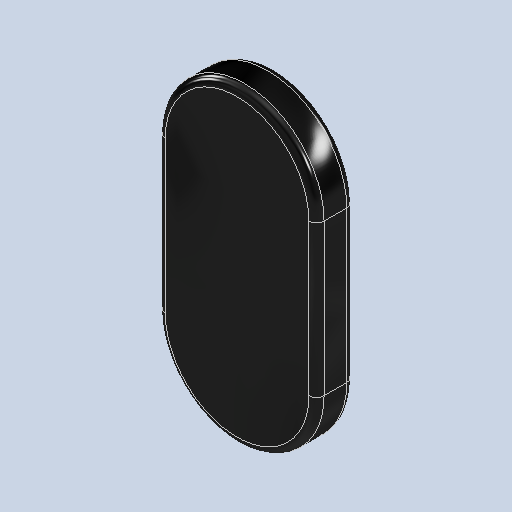
# Autodesk Inventor part: Feets
Saved by Autodesk Inventor 2023.1 (Build 271208000, 208)
## iProperties
Created: 2022-09-12
Part Number: Feets
Material: Generisch
Document SubType Name: Modeling
Designer: Rama
Density: 1 g/cm^3
Appearance: Schwarz
Author: Rama
Autodesk Inventor part; units mm, degrees
ref_plane "YZ Plane" through (0, 0, 0) normal (1, 0, 0) x (0, 1, 0)
ref_plane "XZ Plane" through (0, 0, 0) normal (0, 1, 0) x (-1, 0, 0)
ref_plane "XY Plane" through (0, 0, 0) normal (0, 0, 1) x (1, 0, 0)
sketch "Skizze1" plane through (0, 0, 0) normal (0, 0, 1) x (1, 0, 0)
  arc A0 (3.65, -3.2996) -> (8.25, -3.2996) centre (5.95, -3.2996) ccw projected
  line L0 (8.25, 0.7004) -> (8.25, -3.2996) projected
  arc A1 (8.25, 0.7004) -> (3.65, 0.7004) centre (5.95, 0.7004) ccw projected
  line L1 (3.65, -3.2996) -> (3.65, 0.7004) projected
  line L2 (5.95, -3.2996) -> (5.95, 0.7004) construction
  line L3 (8.05, -3.2996) -> (8.05, 0.7004)
  line L4 (3.85, 0.7004) -> (3.85, -3.2996)
  arc A2 (3.85, -3.2996) -> (8.05, -3.2996) centre (5.95, -3.2996) ccw
  arc A3 (8.05, 0.7004) -> (3.85, 0.7004) centre (5.95, 0.7004) ccw
  point P0 (0, 0)
  point P1 (5.95, -1.2996)
  dimension "d0" = 4.2
  constraints: 8 end point, 4 point on circle, 4 tangent, 2 centre point, 1 midpoint, 1 parallel, 1 vertical
  measures "d0" diameter of A3
extrude "Extrusion1" add sketch "Skizze1" along normal blind 1 contours A2 L4 A3 L3
fillet "Rundung1" radius 0.2 8 edges at (5.95, 2.8004, 1) (3.85, -1.2996, 1) (5.95, -5.3996, 1) (8.05, -1.2996, 1) (5.95, 2.8004, 0) (3.85, -1.2996, 0) (5.95, -5.3996, 0) (8.05, -1.2996, 0)
